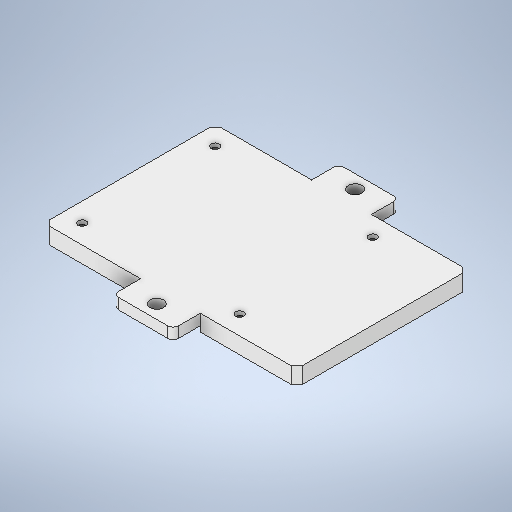
# Autodesk Inventor part: Case Bottom V2
Saved by Autodesk Inventor 2025.2 (Build 292293000, 293)
## iProperties
Created: 2025-04-01
Part Number: Case Bottom V2
Material: PC/ABS Plastic
Document SubType Name: Modeling
Designer: franc
Density: 1.1 g/cm^3
Appearance: Smooth - White
Author: franc
## iProperties of the stored document Case Bottom V2_3DPrint.ipt
Created: 2025-04-12
Part Number: Case Bottom V2_3DPrint
Material: Generic
Document SubType Name: Modeling
Designer: franc
Density: 1 g/cm^3
Appearance: Default
Author: franc
Autodesk Inventor part; units mm, degrees
ref_plane "YZ Plane" through (0, 0, 0) normal (1, 0, 0) x (0, 1, 0)
ref_plane "XZ Plane" through (0, 0, 0) normal (0, 1, 0) x (-1, 0, 0)
ref_plane "XY Plane" through (0, 0, 0) normal (0, 0, 1) x (1, 0, 0)
sketch "Sketch1" plane through (0, 0, 0) normal (0, 1, 0) x (-1, 0, 0)
  line L0 (0, 0) -> (0, 56)
  line L1 (0, 56) -> (-85, 56)
  line L2 (-85, 56) -> (-85, 0)
  line L3 (-85, 0) -> (0, 0)
  circle A0 centre (-3.5, 52.5) radius 1.5
  circle A1 centre (-61.5, 52.5) radius 1.5
  circle A2 centre (-61.5, 3.5) radius 1.5
  circle A3 centre (-3.5, 3.5) radius 1.5
  dimension "d0" = 56
  dimension "d1" = 85
  dimension "d2" = 3
  dimension "d3" = 3.5
  dimension "d4" = 3.5
  dimension "d5" = 3
  dimension "d6" = 3.5
  dimension "d7" = 23.5
  dimension "d8" = 3
  dimension "d9" = 3.5
  dimension "d10" = 23.5
  dimension "d11" = 3
  dimension "d12" = 3.5
  dimension "d13" = 3.5
  constraints: 8 end point, 4 centre point, 2 perpendicular, 1 horizontal, 1 vertical
  measures "d0" distance of L0.start L0.end
  measures "d1" distance of L0.end L1.end
  measures "d2" diameter of A0
  measures "d3" distance from line of A0.centre L0
  measures "d4" distance from line of A0.centre L1
  measures "d5" diameter of A1
  measures "d6" distance from line of L1 A1.centre
  measures "d7" distance from line of A1.centre L2
  measures "d8" diameter of A2
  measures "d9" distance from line of L3 A2.centre
  measures "d10" distance from line of L2 A2.centre
  measures "d11" diameter of A3
  measures "d12" distance from line of L3 A3.centre
  measures "d13" distance from line of L0 A3.centre
extrude "Base - 3.5mm" add sketch "Sketch1" along normal blind 3.5
sketch "Sketch2" plane through (85, 0, 56) normal (1, 0, 0) x (0, 0, -1)
  line L0 (0, 0) -> (56, 0) projected
  line L1 (56, 0) -> (56, 3.5) projected
  line L2 (0, 3.5) -> (56, 3.5) projected
  line L3 (0, 0) -> (0, 3.5) projected
extrude "Extension @ LAN - 4.5mm" add sketch "Sketch2" along normal blind 4.5
sketch "Sketch3" plane through (0, 0, 56) normal (0, 0, 1) x (1, 0, 0)
  line L0 (0, 0) -> (89.5, 0) projected
  line L1 (89.5, 3.5) -> (89.5, 0) projected
  line L2 (0, 3.5) -> (89.5, 3.5) projected
  line L3 (0, 0) -> (0, 3.5) projected
extrude "Extension @ USB - 3.5mm" add sketch "Sketch3" along normal blind 3.5
sketch "Sketch4" plane through (0, 3.5, 0) normal (0, 1, 0) x (1, 0, 0)
  circle A0 centre (3.5, -3.5) radius 1.5 projected
  circle A1 centre (3.5, -3.5) radius 2
  circle A2 centre (3.5, -52.5) radius 1.5 projected
  circle A3 centre (3.5, -52.5) radius 2
  circle A4 centre (61.5, -52.5) radius 1.5 projected
  circle A5 centre (61.5, -52.5) radius 2
  circle A6 centre (61.5, -3.5) radius 1.5 projected
  circle A7 centre (61.5, -3.5) radius 2
  point P0 (0, 0)
  dimension "d21" = 4
  dimension "d22" = 4
  dimension "d23" = 4
  dimension "d24" = 4
  constraints: 4 centre point, 4 coincident
  measures "d21" diameter of A1
  measures "d22" diameter of A3
  measures "d23" diameter of A5
  measures "d24" diameter of A7
extrude "Mount + Spacer Holes - 3.5mm" add sketch "Sketch4" along normal blind 6.8 contours A0 | A1 | A2 | A3 | A4 | A5 | A6 | A7
sketch "Sketch5" plane through (0, 0, 0) normal (0, 0, -1) x (-1, 0, 0)
  line L0 (0, 0) -> (-89.5, 0) projected
  line L1 (0, 0) -> (0, 3.5) projected
  line L2 (0, 3.5) -> (-89.5, 3.5) projected
  line L3 (-89.5, 0) -> (-89.5, 3.5) projected
extrude "GPIO Side - 3.5mm" add sketch "Sketch5" along normal blind 3.5
sketch "Sketch6" plane through (0, 0, 59.5) normal (-1, 0, 0) x (0, 0, 1)
  line L0 (0, 0) -> (-63, 0) projected
  line L1 (0, 3.5) -> (0, 0) projected
  line L2 (0, 3.5) -> (-63, 3.5) projected
  line L3 (-63, 0) -> (-63, 3.5) projected
  point P0 (-59.5, 0)
extrude "Power Button side - 3.5mm" add sketch "Sketch6" along normal blind 3.5
chamfer "Edges Chamfer - 2mm" distance 2 angle 45 4 edges at (89.5, 1.75, 59.5) (89.5, 1.75, -3.5) (-3.5, 1.75, -3.5) (-3.5, 1.75, 59.5)
sketch "Sketch8" plane through (0, 0, 59.5) normal (0, 0, 1) x (1, 0, 0)
  line L0 (43, 1) -> (33, 1)
  line L1 (33, 0) -> (33, -2.5)
  line L2 (33, -2.5) -> (32, -2.5)
  line L3 (32, -2.5) -> (32, 3.5)
  line L4 (87.5, 3.5) -> (-1.5, 3.5) projected
  line L5 (43, 1) -> (53, 1)
  line L6 (53, 0) -> (53, -2.5)
  line L7 (53, -2.5) -> (54, -2.5)
  line L8 (54, -2.5) -> (54, 3.5)
  line L9 (32, 3.5) -> (54, 3.5)
  line L10 (33, 0) -> (53, 0)
  point P0 (0, 0)
  dimension "d48" = 10
  dimension "d50" = 1
  dimension "d52" = 1
  constraints: 20 end point, 4 perpendicular, 4 point on line, 1 collinear
  measures "d48" distance of L0.start L0.end
  measures "d50" distance of L1.end L2.end
  measures "d52" distance of L6.end L7.end
extrude "Mounting Guides" add sketch "Sketch8" along normal blind 10 and the other way blind 1
sketch "Sketch9" plane through (0, 0, -3.5) normal (0, 0, -1) x (-1, 0, 0)
  line L0 (-54, 3.5) -> (-54, 0) projected
  line L1 (-54, 1) -> (-54, 0) projected
  line L2 (-54, 0) -> (-54, -2.5) projected
  line L3 (-54, -2.5) -> (-53, -2.5) projected
  line L4 (-53, -2.5) -> (-53, 0) projected
  line L5 (-87.0858, 0) -> (1.0858, 0) projected
  line L6 (-33, 0) -> (-33, -2.5) projected
  line L7 (-33, -2.5) -> (-32, -2.5) projected
  line L8 (-32, -2.5) -> (-32, 0) projected
  line L9 (-32, 0) -> (-32, 3.5) projected
  line L10 (-32, 0) -> (-32, 1) projected
  line L11 (-87.5, 3.5) -> (1.5, 3.5) projected
  point P0 (0, 0)
extrude "Extrusion9" add sketch "Sketch9" along normal blind 10 and the other way blind 1
sketch "Sketch10" plane through (0, 3.5, 0) normal (0, 1, 0) x (1, 0, 0)
  line L0 (33, -69.5) -> (53, -69.5) projected
  line L1 (53, 13.5) -> (33, 13.5) projected
  line L2 (54, -69.5) -> (32, -69.5) projected
  circle A0 centre (43, -64.5) radius 2.5
  circle A1 centre (43, 8.5) radius 2.5
  point P0 (0, 0)
  point P1 (43, -69.5)
  point P2 (43, 13.5)
  dimension "d63" = 5
  dimension "d64" = 5
  dimension "d65" = 5
  constraints: 2 centre point, 2 midpoint
  measures "d63" diameter of A0
  measures "d64" diameter of A1
  measures "d65" distance from line of L1 A1.centre
extrude "Extrusion10" cut sketch "Sketch10" against normal through all
sketch "Sketch13" plane through (0, 0, 69.5) normal (0, 0, 1) x (1, 0, 0)
  line L0 (33, -2.5) -> (32, -2.5) projected
  line L1 (32, -2.5) -> (54, -2.5)
  line L2 (54, -2.5) -> (54, 0)
  line L3 (54, 0) -> (32, 0)
  line L4 (32, 0) -> (32, -2.5)
  point P0 (0, 0)
  constraints: 8 end point, 2 parallel, 1 horizontal, 1 perpendicular
extrude "Extrusion13" cut sketch "Sketch13" against normal through all
sketch "Sketch15" plane through (61.5, 3.5, 3.5) normal (0, -1, 0) x (1, 0, 0)
  circle A0 centre (0, 0) radius 1.5 projected
  circle A1 centre (-58, 0) radius 1.5 projected
  circle A2 centre (0, 49) radius 1.5 projected
  circle A3 centre (-58, 49) radius 1.5 projected
  point P0 (-61.5, -3.5)
extrude "Extrusion14" add sketch "Sketch15" along normal up to surface (3.5 mm away)
sketch "Sketch16" plane through (61.5, 10.3, 3.5) normal (0, 1, 0) x (1, 0, 0)
  circle A0 centre (-58, 0) radius 2 projected
  circle A1 centre (-58, 0) radius 1.25
  circle A2 centre (0, 0) radius 2 projected
  circle A3 centre (0, 0) radius 1.25
  circle A4 centre (0, -49) radius 2 projected
  circle A5 centre (0, -49) radius 1.25
  circle A6 centre (-58, -49) radius 2 projected
  circle A7 centre (-58, -49) radius 1.25
  point P0 (-61.5, 3.5)
  dimension "d79" = 2.5
  dimension "d80" = 2.5
  dimension "d81" = 2.5
  dimension "d82" = 2.5
  constraints: 4 centre point, 4 coincident
  measures "d79" diameter of A1
  measures "d80" diameter of A3
  measures "d81" diameter of A5
  measures "d82" diameter of A7
extrude "Extrusion15" add sketch "Sketch16" along normal blind 5 and the other way blind 6.8 contours A1 | A3 | A5 | A7
sketch "Sketch18" plane through (3.5, 15.3, 52.5) normal (0, 1, 0) x (1, 0, 0)
  circle A0 centre (0, 49) radius 2 projected
  circle A1 centre (58, 49) radius 2 projected
  circle A2 centre (58, 0) radius 2 projected
  circle A3 centre (0, 0) radius 2 projected
  point P0 (-3.5, 52.5)
extrude "Extrusion16" cut sketch "Sketch18" against normal through all
sketch "Sketch19" plane through (0, 3.5, 0) normal (0, 1, 0) x (1, 0, 0)
  circle A0 centre (43, 8.5) radius 2.5 projected
  circle A1 centre (43, -64.5) radius 2.5 projected
  circle A2 centre (3.5, -52.5) radius 2 projected
  circle A3 centre (3.5, -3.5) radius 2 projected
  circle A4 centre (61.5, -52.5) radius 2 projected
  circle A5 centre (61.5, -3.5) radius 2 projected
  line L0 (32, 3.5) -> (-1.5, 3.5) projected
  line L1 (-3.5, 1.5) -> (-1.5, 3.5) projected
  line L2 (-3.5, -57.5) -> (-3.5, 1.5) projected
  line L3 (-1.5, -59.5) -> (-3.5, -57.5) projected
  line L4 (32, -59.5) -> (-1.5, -59.5) projected
  line L5 (32, -59.5) -> (32, -69.5) projected
  line L6 (54, -69.5) -> (32, -69.5) projected
  line L7 (54, -59.5) -> (54, -69.5) projected
  line L8 (87.5, -59.5) -> (54, -59.5) projected
  line L9 (89.5, -57.5) -> (87.5, -59.5) projected
  line L10 (89.5, -57.5) -> (89.5, 1.5) projected
  line L11 (87.5, 3.5) -> (89.5, 1.5) projected
  line L12 (87.5, 3.5) -> (54, 3.5) projected
  line L13 (54, 3.5) -> (54, 13.5) projected
  line L14 (32, 13.5) -> (54, 13.5) projected
  line L15 (32, 3.5) -> (32, 13.5) projected
  point P0 (0, 0)
extrude "Extrusion17" add sketch "Sketch19" along normal blind 2.5
sketch "Sketch20" plane through (0, 0, 0) normal (0, -1, 0) x (1, 0, 0)
  circle A0 centre (3.5, 52.5) radius 2 projected
  line L0 (3.5, 49.5) -> (0.9019, 51)
  line L1 (0.9019, 51) -> (0.9019, 54)
  line L2 (0.9019, 54) -> (3.5, 55.5)
  line L3 (3.5, 55.5) -> (6.0981, 54)
  line L4 (6.0981, 54) -> (6.0981, 51)
  line L5 (6.0981, 51) -> (3.5, 49.5)
  circle A1 centre (61.5, 52.5) radius 2 projected
  line L6 (61.5, 49.5) -> (58.9019, 51)
  line L7 (58.9019, 51) -> (58.9019, 54)
  line L8 (58.9019, 54) -> (61.5, 55.5)
  line L9 (61.5, 55.5) -> (64.0981, 54)
  line L10 (64.0981, 54) -> (64.0981, 51)
  line L11 (64.0981, 51) -> (61.5, 49.5)
  circle A2 centre (61.5, 3.5) radius 2 projected
  line L12 (64.0981, 2) -> (61.5, 0.5)
  line L13 (61.5, 0.5) -> (58.9019, 2)
  line L14 (58.9019, 2) -> (58.9019, 5)
  line L15 (58.9019, 5) -> (61.5, 6.5)
  line L16 (61.5, 6.5) -> (64.0981, 5)
  line L17 (64.0981, 5) -> (64.0981, 2)
  line L18 (6.0981, 2) -> (3.5, 0.5)
  line L19 (3.5, 0.5) -> (0.9019, 2)
  line L20 (0.9019, 2) -> (0.9019, 5)
  line L21 (0.9019, 5) -> (3.5, 6.5)
  line L22 (3.5, 6.5) -> (6.0981, 5)
  line L23 (6.0981, 5) -> (6.0981, 2)
  point P0 (0, 0)
  point P1 (3.5, 3.5)
  point P2 (3.5, 3.5)
  dimension "d107" = 3
  constraints: 48 end point, 4 coincident, 52 other
  measures "d107" distance of A0.centre L0.start
extrude "Extrusion18" cut sketch "Sketch20" against normal blind 4.5
sketch "Sketch21" plane through (0, 6, 0) normal (0, 1, 0) x (1, 0, 0)
  circle A0 centre (3.5, -3.5) radius 2 projected
  circle A1 centre (3.5, -3.5) radius 1.5
  circle A2 centre (3.5, -52.5) radius 2 projected
  circle A3 centre (3.5, -52.5) radius 1.5
  circle A4 centre (61.5, -52.5) radius 2 projected
  circle A5 centre (61.5, -52.5) radius 1.5
  circle A6 centre (61.5, -3.5) radius 2 projected
  circle A7 centre (61.5, -3.5) radius 1.5
  point P0 (0, 0)
  dimension "d95" = 3
  dimension "d96" = 3
  dimension "d97" = 3
  dimension "d98" = 3
  constraints: 4 centre point, 4 coincident
  measures "d95" diameter of A1
  measures "d96" diameter of A3
  measures "d97" diameter of A5
  measures "d98" diameter of A7
extrude "Extrusion19" add sketch "Sketch21" against normal up to surface (1.5 mm away)
fillet "Fillet5" radius 2 4 edges at (54, 3, -13.5) (32, 3, -13.5) (54, 3, 69.5) (32, 3, 69.5)
sketch "Sketch24" plane through (0, 0, 0) normal (0, -1, 0) x (1, 0, 0)
  line L0 (87.5, -3.5) -> (54, -3.5) projected
  line L1 (54, -3.5) -> (54, 59.5)
  line L2 (32, -3.5) -> (-1.5, -3.5) projected
  line L3 (32, -3.5) -> (32, 59.5)
  line L4 (54, 67.5) -> (54, 59.5) projected
  line L5 (34, 69.5) -> (52, 69.5) projected
  arc A0 (54, 67.5) -> (52, 69.5) centre (52, 67.5) ccw projected
  arc A1 (34, 69.5) -> (32, 67.5) centre (34, 67.5) ccw projected
  line L6 (32, 59.5) -> (32, 67.5) projected
  circle A2 centre (43, 64.5) radius 2.5 projected
  line L7 (54, -3.5) -> (54, -11.5) projected
  arc A3 (52, -13.5) -> (54, -11.5) centre (52, -11.5) ccw projected
  line L8 (52, -13.5) -> (34, -13.5) projected
  circle A4 centre (43, -8.5) radius 2.5 projected
  arc A5 (32, -11.5) -> (34, -13.5) centre (34, -11.5) ccw projected
  line L9 (32, -11.5) -> (32, -3.5) projected
  point P0 (0, 0)
  constraints: 4 end point
extrude "Extrusion21" cut sketch "Sketch24" against normal blind 2
body "Solid1"
